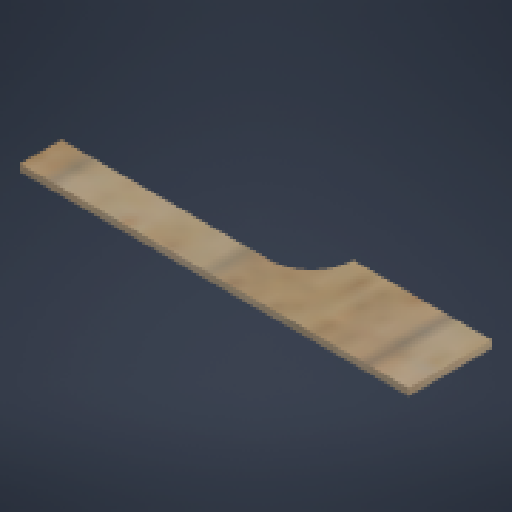
# Autodesk Inventor part: base
Saved by Autodesk Inventor 2026.1 (Build 301233020, 233B)
## iProperties
Created: 2025-09-27
Part Number: base
Material: 木材 (カエデ材)
Document SubType Name: Modeling
Designer: hibik
Density: 0.67 g/cm^3
Appearance: ナチュラル カエデ材 - 光沢 濃い着色
Author: hibik
Autodesk Inventor part; units mm, degrees
ref_plane "YZ Plane" through (0, 0, 0) normal (1, 0, 0) x (0, 1, 0)
ref_plane "XZ Plane" through (0, 0, 0) normal (0, 1, 0) x (-1, 0, 0)
ref_plane "XY Plane" through (0, 0, 0) normal (0, 0, 1) x (1, 0, 0)
sketch "スケッチ1" plane through (0, 0, 0) normal (0, 1, 0) x (-1, 0, 0)
  line L0 (0, 99) -> (140, 99)
  line L1 (140, -99) -> (0, -99)
  line L2 (0, -99) -> (0, 99)
  line L3 (20, 99) -> (20, -99)
  line L4 (140, 99) -> (140, -99)
  line L5 (50, 99) -> (50, -99)
  line L6 (140, 84) -> (50, 84)
  line L7 (50, 69) -> (0, 69)
  point P0 (0, 0)
  point P1 (0, 0)
  point P2 (0, 69)
  dimension "d0" = 198
  dimension "d3" = 20
  dimension "d4" = 120
  dimension "d30" = 30
  dimension "d31" = 15
  dimension "d33" = 30
  constraints: 16 end point, 12 point on line, 2 horizontal, 2 perpendicular, 2 vertical, 1 coincident, 1 midpoint, 1 parallel
  measures "d0" distance of L0.end L1.start
  measures "d3" distance between parallel lines of L2 L3
  measures "d4" distance between parallel lines of L3 L4
  measures "d30" distance between parallel lines of L3 L5
  measures "d31" distance between parallel lines of L0 L6
  measures "d33" distance between parallel lines of L0 L7
extrude "押し出し1" add sketch "スケッチ1" along normal blind 2.5 contours L0 L3 L7 L2 | L0 L5 L7 L3 | L0 L4 L6 L5
fillet "フィレット2" radius 15 1 edges at (-50, 1.25, 84)
